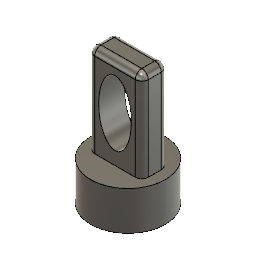
Ladle Loop (Autodesk Fusion 360 design; units mm, degrees)
Autodesk Fusion 360 part; units mm, degrees
sketch "Sketch1" plane through (0, 0, 0) normal (0, 1, 0) x (1, 0, 0)
  circle A0 centre (0, 0) radius 8.1
  circle A1 centre (0, 0) radius 11.5
  dimension "d1" = 16.2
  dimension "d2" = 23
  constraint coincident A0.centre A1.centre
  constraint concentric A0 A1
  measures "d1" diameter of A0
  measures "d2" diameter of A1
extrude "Extrude1" add sketch "Sketch1" along normal blind 10
extrude "Extrude2" add sketch "Sketch1" along normal blind 2 from surface at 10 contours A0 | A1
sketch "Sketch2" plane through (0, 0, 0) normal (0, 0, 1) x (1, 0, 0)
  ellipse E0 centre (0, 26) end of major axis (0, 36) minor radius 5
  line L0 (0, 16) -> (0, 36)
  line L1 (5, 26) -> (-5, 26)
  dimension "d8" = 20
  dimension "d9" = 10
  dimension "d10" = 26
  constraint coincident E0 L0.start
  constraint coincident E0 L0.end
  constraint coincident E0 L1.start
  constraint coincident E0 L1.end
  constraint vertical origin E0.centre
  measures "d8" distance of E0
  measures "d9" distance of E0
  measures "d10" distance of origin E0.centre
sketch "Sketch3" plane through (0, 0, 0) normal (0, 0, 1) x (1, 0, 0)
  line L0 (8.25, 12) -> (-8.25, 12)
  line L1 (-8.25, 12) -> (-8.25, 40)
  line L2 (-8.25, 40) -> (8.25, 40)
  line L3 (8.25, 40) -> (8.25, 12)
  line L4 (8.25, 12) -> (-8.25, 40) construction
  line L5 (-8.25, 12) -> (8.25, 40) construction
  point P0 (0, 26)
  dimension "d11" = 16.5
  dimension "d12" = 28
  dimension "d13" = 12
  constraint perpendicular L0 L1
  constraint parallel L0 L2
  constraint parallel L1 L3
  constraint horizontal L0
  constraint coincident L4 P0
  constraint coincident L5 P0
  constraint vertical origin P0
  measures "d11" distance of L1.end L2.end
  measures "d12" distance of L0.end L1.end
  measures "d13" distance of L0 origin
extrude "Extrude3" add sketch "Sketch3" along normal mid plane 8
extrude "Extrude4" cut sketch "Sketch2" along normal mid plane 20
fillet "Fillet1" radius 2 8 edges at (8.25, 26, 4) (8.25, 26, -4) (0, 40, 4) (0, 40, -4) (8.25, 40, 0) (-8.25, 40, 0) (-8.25, 26, 4) (-8.25, 26, -4)
